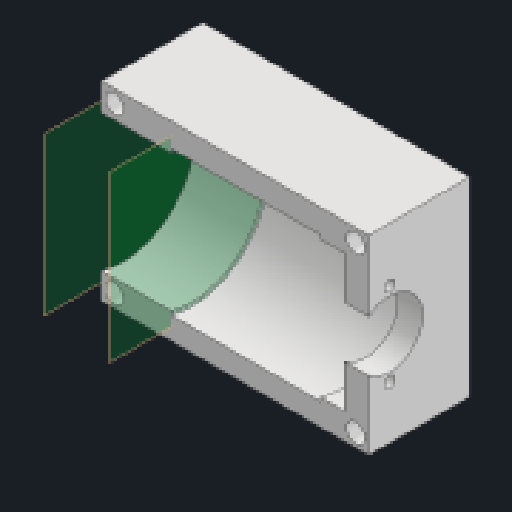
# Autodesk Inventor part: motor_mount_right
Saved by Autodesk Inventor 2023 (Build 270158000, 158)
## iProperties
Created: 2024-04-14
Part Number: motor_mount_right
Material: Generic
Document SubType Name: Modeling
Designer: szymo
Density: 1 g/cm^3
Appearance: Default
Author: szymo
Autodesk Inventor part; units mm, degrees
ref_plane "YZ Plane" through (0, 0, 0) normal (1, 0, 0) x (0, 1, 0)
ref_plane "XZ Plane" through (0, 0, 0) normal (0, 1, 0) x (-1, 0, 0)
ref_plane "XY Plane" through (0, 0, 0) normal (0, 0, 1) x (1, 0, 0)
ref_plane "Work Plane1" through (-73.7, 19.125, 15.375) normal (-1, 0, 0) x (0, 1, 0)
sketch "Sketch1" plane through (-73.7, 19.125, 15.375) normal (-1, 0, 0) x (0, 1, 0)
  line L0 (18.375, 18.375) -> (-92.625, 18.375) projected
  line L1 (-92.625, 18.375) -> (-92.625, 15.375) projected
  line L2 (18.375, 15.375) -> (-92.625, 15.375) projected
  line L3 (18.375, 18.375) -> (18.375, 15.375) projected
  line L4 (11, 1.5) -> (11.5, 1.5) projected
  line L5 (11.5, 1.5) -> (11.5, -1.5) projected
  line L6 (11.5, -1.5) -> (11, -1.5) projected
  line L7 (11, -1.5) -> (11, 1.5) projected
  line L8 (-11.5, -1.5) -> (-12, -1.5) projected
  line L9 (-12, -1.5) -> (-12, 1.5) projected
  line L10 (-12, 1.5) -> (-11.5, 1.5) projected
  line L11 (-11.5, 1.5) -> (-11.5, -1.5) projected
  circle A0 centre (0, 0) radius 5 projected
  circle A1 centre (0, 0) radius 13.7 projected
  line L12 (18.375, 15.375) -> (-18.1, 15.375)
  line L13 (-18.1, 15.375) -> (-18.1, -4)
  line L14 (-18.1, -4) -> (18.375, -4)
  line L15 (18.375, -4) -> (18.375, 15.375)
  point P0 (-19.125, 15.375)
  point P1 (-13.7, 0)
  point P2 (13.7, 0)
  point P3 (-18.1, 15.375)
  point P4 (-13.1031, -4)
  point P5 (13.1031, -4)
  dimension "d0" = 4
  dimension "d2" = 15.375
  dimension "d3" = 15.375
  dimension "d4" = 4.675
  dimension "d5" = 4.4
  constraints: 8 end point, 2 parallel, 2 point on circle, 1 horizontal, 1 perpendicular
  measures "d0" distance from line of L14 A0.centre
  measures "d2" distance from line of L2 A1.end
  measures "d3" distance from line of L12 A1.start
  measures "d4" distance from line of L15 A1.end
  measures "d5" distance from line of A1.start L13
ref_plane "Work Plane2" through (-27.2, 5.425, 1.675) normal (1, 0, 0) x (0, 1, 0)
extrude "Extrusion1" add sketch "Sketch1" against normal up to surface (46.5 mm away) contours L15 L14 A1 L13 L2
sketch "Sketch2" plane through (-27.2, 19.125, 15.375) normal (1, 0, 0) x (0, 0, -1)
  circle A0 centre (0, -8) radius 1.0564 projected
  circle A1 centre (0, 8) radius 1.0564 projected
  circle A2 centre (0, 0) radius 5 projected
  circle A3 centre (0, 0) radius 13.7 projected
  line L0 (18.375, 18.375) -> (18.375, -91.625) projected
  arc A4 (1.3629, -5.6821) -> (1.478, -3.5703) centre (-3.2424, -4.3721) ccw projected
  arc A5 (1.478, -3.5703) -> (2.0183, -3.2951) centre (0, 0) ccw projected
  arc A6 (2.0183, -3.2951) -> (3.794, -4.444) centre (5.443, 0.0511) ccw projected
  arc A7 (3.794, -4.444) -> (4.4425, -3.7958) centre (0, 0) ccw projected
  arc A8 (4.4425, -3.7958) -> (3.2943, -2.0197) centre (-0.0533, -5.443) ccw projected
  arc A9 (3.2943, -2.0197) -> (3.5697, -1.4795) centre (0, 0) ccw projected
  arc A10 (3.5697, -1.4795) -> (5.6815, -1.3652) centre (4.3734, 3.2407) ccw projected
  arc A11 (5.6815, -1.3652) -> (5.8252, -0.4596) centre (0, 0) ccw projected
  arc A12 (5.8252, -0.4596) -> (3.8523, 0.3024) centre (3.1561, -4.4348) ccw projected
  arc A13 (3.8523, 0.3024) -> (3.7575, 0.9013) centre (0, 0) ccw projected
  arc A14 (3.7575, 0.9013) -> (5.3989, 2.235) centre (1.6334, 5.1924) ccw projected
  arc A15 (5.3989, 2.235) -> (4.9828, 3.0521) centre (0, 0) ccw projected
  arc A16 (4.9828, 3.0521) -> (2.9388, 2.5089) centre (5.1601, -1.7327) ccw projected
  arc A17 (2.9388, 2.5089) -> (2.5101, 2.9378) centre (0, 0) ccw projected
  arc A18 (2.5101, 2.9378) -> (3.0541, 4.9816) centre (-1.7306, 5.1608) ccw projected
  arc A19 (3.0541, 4.9816) -> (2.2372, 5.398) centre (0, 0) ccw projected
  arc A20 (2.2372, 5.398) -> (0.9028, 3.7572) centre (5.193, 1.6313) ccw projected
  arc A21 (0.9028, 3.7572) -> (0.304, 3.8521) centre (0, 0) ccw projected
  arc A22 (0.304, 3.8521) -> (-0.4573, 5.8253) centre (-4.4335, 3.1579) ccw projected
  arc A23 (-0.4573, 5.8253) -> (-1.3629, 5.6821) centre (0, 0) ccw projected
  arc A24 (-1.3629, 5.6821) -> (-1.478, 3.5703) centre (3.2424, 4.3721) ccw projected
  arc A25 (-1.478, 3.5703) -> (-2.0183, 3.2951) centre (0, 0) ccw projected
  arc A26 (-2.0183, 3.2951) -> (-3.794, 4.444) centre (-5.443, -0.0511) ccw projected
  arc A27 (-3.794, 4.444) -> (-4.4425, 3.7958) centre (0, 0) ccw projected
  arc A28 (-4.4425, 3.7958) -> (-3.2943, 2.0197) centre (0.0533, 5.443) ccw projected
  arc A29 (-3.2943, 2.0197) -> (-3.5697, 1.4795) centre (0, 0) ccw projected
  arc A30 (-3.5697, 1.4795) -> (-5.6815, 1.3652) centre (-4.3734, -3.2407) ccw projected
  arc A31 (-5.6815, 1.3652) -> (-5.8252, 0.4596) centre (0, 0) ccw projected
  arc A32 (-5.8252, 0.4596) -> (-3.8523, -0.3024) centre (-3.1561, 4.4348) ccw projected
  arc A33 (-3.8523, -0.3024) -> (-3.7575, -0.9013) centre (0, 0) ccw projected
  arc A34 (-3.7575, -0.9013) -> (-5.3989, -2.235) centre (-1.6334, -5.1924) ccw projected
  arc A35 (-5.3989, -2.235) -> (-4.9828, -3.0521) centre (0, 0) ccw projected
  arc A36 (-4.9828, -3.0521) -> (-2.9388, -2.5089) centre (-5.1601, 1.7327) ccw projected
  arc A37 (-2.9388, -2.5089) -> (-2.5101, -2.9378) centre (0, 0) ccw projected
  arc A38 (-2.5101, -2.9378) -> (-3.0541, -4.9816) centre (1.7306, -5.1608) ccw projected
  arc A39 (-3.0541, -4.9816) -> (-2.2372, -5.398) centre (0, 0) ccw projected
  arc A40 (-2.2372, -5.398) -> (-0.9028, -3.7572) centre (-5.193, -1.6313) ccw projected
  arc A41 (-0.9028, -3.7572) -> (-0.304, -3.8521) centre (0, 0) ccw projected
  arc A42 (-0.304, -3.8521) -> (0.4573, -5.8253) centre (4.4335, -3.1579) ccw projected
  arc A43 (0.4573, -5.8253) -> (1.3629, -5.6821) centre (0, 0) ccw projected
  line L1 (15.375, -18.1) -> (-4, -18.1) projected
  line L2 (15.375, 18.375) -> (15.375, -18.1) projected
  line L3 (-4, 18.375) -> (15.375, 18.375) projected
  line L4 (-4, 13.1031) -> (-4, 18.375) projected
  arc A44 (-4, -13.1031) -> (-4, 13.1031) centre (0, 0) ccw projected
  line L5 (-4, -18.1) -> (-4, -13.1031) projected
  line L6 (-4, -18.1) -> (-4, -13.1031) projected
  line L7 (15.375, 18.375) -> (15.375, -18.1) projected
  line L8 (-4, -18.1) -> (15.375, -18.1)
  line L9 (15.375, -18.1) -> (15.375, 18.375)
  line L10 (15.375, 18.375) -> (-4, 18.375)
  line L11 (-4, 18.375) -> (-4, -18.1)
  circle A45 centre (0, -8) radius 1.0564
  circle A46 centre (0, 8) radius 1.0564
  arc A47 (6.0944, -1.7595) -> (6.3397, -0.2124) centre (0, 0) ccw
  arc A48 (3.9887, -2.0334) -> (6.0944, -1.7595) centre (4.3734, 3.2407) ccw
  arc A49 (5.0041, -3.8982) -> (3.9887, -2.0334) centre (-0.0533, -5.443) ccw
  arc A50 (3.8962, -5.0057) -> (5.0041, -3.8982) centre (0, 0) ccw
  arc A51 (2.0318, -3.9896) -> (3.8962, -5.0057) centre (5.443, 0.0511) ccw
  arc A52 (1.7571, -6.0951) -> (2.0318, -3.9896) centre (-3.2424, -4.3721) ccw
  arc A53 (0.2098, -6.3398) -> (1.7571, -6.0951) centre (0, 0) ccw
  arc A54 (-0.7013, -4.4219) -> (0.2098, -6.3398) centre (4.4335, -3.1579) ccw
  arc A55 (-2.1611, -5.9638) -> (-0.7013, -4.4219) centre (-5.193, -1.6313) ccw
  arc A56 (-3.5567, -5.2523) -> (-2.1611, -5.9638) centre (0, 0) ccw
  arc A57 (-3.1665, -3.1652) -> (-3.5567, -5.2523) centre (1.7306, -5.1608) ccw
  arc A58 (-5.2538, -3.5545) -> (-3.1665, -3.1652) centre (-5.1601, 1.7327) ccw
  arc A59 (-5.9647, -2.1587) -> (-5.2538, -3.5545) centre (0, 0) ccw
  arc A60 (-4.4222, -0.6995) -> (-5.9647, -2.1587) centre (-1.6334, -5.1924) ccw
  arc A61 (-6.3397, 0.2124) -> (-4.4222, -0.6995) centre (-3.1561, 4.4348) ccw
  arc A62 (-6.0944, 1.7595) -> (-6.3397, 0.2124) centre (0, 0) ccw
  arc A63 (-3.9887, 2.0334) -> (-6.0944, 1.7595) centre (-4.3734, -3.2407) ccw
  arc A64 (-5.0041, 3.8982) -> (-3.9887, 2.0334) centre (0.0533, 5.443) ccw
  arc A65 (-3.8962, 5.0057) -> (-5.0041, 3.8982) centre (0, 0) ccw
  arc A66 (-2.0318, 3.9896) -> (-3.8962, 5.0057) centre (-5.443, -0.0511) ccw
  arc A67 (-1.7571, 6.0951) -> (-2.0318, 3.9896) centre (3.2424, 4.3721) ccw
  arc A68 (-0.2098, 6.3398) -> (-1.7571, 6.0951) centre (0, 0) ccw
  arc A69 (0.7013, 4.4219) -> (-0.2098, 6.3398) centre (-4.4335, 3.1579) ccw
  arc A70 (2.1611, 5.9638) -> (0.7013, 4.4219) centre (5.193, 1.6313) ccw
  arc A71 (3.5567, 5.2523) -> (2.1611, 5.9638) centre (0, 0) ccw
  arc A72 (3.1665, 3.1652) -> (3.5567, 5.2523) centre (-1.7306, 5.1608) ccw
  arc A73 (5.2538, 3.5545) -> (3.1665, 3.1652) centre (5.1601, -1.7327) ccw
  arc A74 (5.9647, 2.1587) -> (5.2538, 3.5545) centre (0, 0) ccw
  arc A75 (4.4222, 0.6995) -> (5.9647, 2.1587) centre (1.6334, 5.1924) ccw
  arc A76 (6.3397, -0.2124) -> (4.4222, 0.6995) centre (3.1561, -4.4348) ccw
  circle A77 centre (0, 0) radius 6.3433
  point P0 (15.375, -19.125)
  point P1 (-4, 13.1031)
  point P2 (-4, 4.9231)
  point P3 (-3.8962, 5.0057)
  point P4 (-1.7571, 6.0951)
  point P5 (-0.2098, 6.3398)
  point P6 (2.1611, 5.9638)
  point P7 (3.5567, 5.2523)
  point P8 (5.2538, 3.5545)
  point P9 (5.9647, 2.1587)
  point P10 (6.3397, -0.2124)
  point P11 (5.0041, -3.8982)
  point P12 (3.8962, -5.0057)
  point P13 (1.7571, -6.0951)
  point P14 (0.2098, -6.3398)
  point P15 (-2.1611, -5.9638)
  point P16 (-3.5567, -5.2523)
  point P17 (-4, -4.9231)
  dimension "d8" = 0.5
  constraints: 60 point on circle, 32 centre point, 8 end point, 3 coincident, 2 concentric, 2 parallel, 1 horizontal, 1 perpendicular, 32 other
  measures "d8" radial gap between concentric circles of A11 A47
ref_plane "Work Plane3" through (-22.5, 37.5, -3) normal (-1, 0, 0) x (0, 0, 1)
extrude "Extrusion2" add sketch "Sketch2" along normal up to surface (4.7 mm away) contours A77 A74 A71 A68 A65 L11 A3 A56 A53 A50 A47 | L4 L3 L2 L1 L5 A3
sketch "Sketch3" plane through (-73.7, 32.2281, 19.375) normal (0, 0, 1) x (1, 0, 0)
  line L0 (0, 5.2719) -> (51.2, 5.2719) projected
  line L1 (0, 0) -> (0, 5.2719) projected
  line L2 (0, 0) -> (46.5, 0) projected
  line L3 (46.5, 0) -> (46.5, -8.1799) projected
  line L4 (46.5, -8.1799) -> (51.2, -8.1799) projected
  line L5 (51.2, 5.2719) -> (51.2, -8.1799) projected
  line L6 (0, -26.2061) -> (46.5, -26.2061) projected
  line L7 (0, -31.2031) -> (0, -26.2061) projected
  line L8 (0, -31.2031) -> (51.2, -31.2031) projected
  line L9 (51.2, -18.0262) -> (51.2, -31.2031) projected
  line L10 (46.5, -18.0262) -> (51.2, -18.0262) projected
  line L11 (46.5, -18.0262) -> (46.5, -26.2061) projected
  line L12 (2.5, 2.7719) -> (48.7, 2.7719)
  line L13 (48.7, 2.7719) -> (48.7, -28.7031)
  line L14 (48.7, -28.7031) -> (2.5, -28.7031)
  line L15 (2.5, -28.7031) -> (2.5, 2.7719)
  point P0 (73.7, -32.2281)
  dimension "d11" = 2.5
  dimension "d12" = 2.5
  dimension "d13" = 2.5
  dimension "d14" = 2.5
  constraints: 8 end point, 4 coincident, 2 parallel, 1 horizontal, 1 perpendicular
  measures "d11" distance between parallel lines of L0 L12
  measures "d12" distance between parallel lines of L5 L13
  measures "d13" distance between parallel lines of L8 L14
  measures "d14" distance between parallel lines of L7 L15
hole "Hole1" at (-71.2, 3.525, 19.375) at (-71.2, 35, 19.375) at (-25, 35, 19.375) at (-25, 3.525, 19.375) direction (0, 0, -1) diameter 3.6 end through all counterbore diameter 11 counterbore depth 0 clearance for "Hex Head Cap Screw ISO 24017" size "M3" standard "ISO"
ref_plane "Work Plane4" through (-60.4, 19.125, 15.375) normal (-1, 0, 0) x (0, 1, 0)
sketch "Sketch4" plane through (-60.4, 19.125, 15.375) normal (-1, 0, 0) x (0, 1, 0)
  circle A0 centre (0, 0) radius 14.375 projected
  point P0 (-19.125, 15.375)
extrude "Extrusion3" cut sketch "Sketch4" against normal blind 28.7
body "Solid1"
